Autodesk Fusion 360 part; units mm, degrees
(part 4 of 7)
  line L2251 (-109.1951, 81.084) -> (-109.1951, 80.0836)
  line L2252 (176.267, 48.0333) -> (162.267, 48.0333)
  line L2253 (200.082, 29.9838) -> (200.879, 29.9838)
  line L2254 (-109.9941, 71.1844) -> (-109.9941, 68.0838)
  line L2255 (204.329, 38.8844) -> (205.13, 38.8844)
  line L2256 (-9.983, 22.9336) -> (-9.183, 22.9336)
  line L2257 (219.132, 19.8345) -> (219.132, 14.0343)
  line L2258 (204.329, 41.9836) -> (205.13, 41.9836)
  line L2259 (224.18, 9.9333) -> (224.18, 10.9337)
  line L2260 (219.929, 14.0343) -> (219.132, 14.0343)
  line L2261 (43.205, 71.1844) -> (42.406, 71.1844)
  line L2262 (-109.9941, 68.0838) -> (-109.9941, 71.1844)
  line L2263 (223.379, 10.9337) -> (224.18, 10.9337)
  line L2264 (204.329, 14.0343) -> (205.13, 14.0343)
  line L2265 (4.817, 23.934) -> (-9.183, 23.934)
  line L2266 (200.879, 10.9337) -> (200.082, 10.9337)
  line L2267 (0.342, 28.9833) -> (14.342, 28.9833)
  line L2268 (200.879, 29.9838) -> (200.879, 33.0844)
  line L2269 (195.605, 0.1836) -> (195.605, 0.7845)
  line L2270 (219.132, 22.9336) -> (219.132, 23.934)
  line L2271 (-109.1951, 76.9844) -> (-109.1951, 71.1844)
  line L2272 (223.379, 14.0343) -> (224.18, 14.0343)
  line L2273 (-109.9941, 76.9844) -> (-109.1951, 76.9844)
  line L2274 (200.082, 10.9337) -> (200.082, 9.9333)
  line L2275 (23.867, 23.934) -> (9.867, 23.934)
  line L2276 (200.082, 9.9333) -> (200.082, 10.9337)
  line L2277 (224.18, 22.9336) -> (223.379, 22.9336)
  line L2278 (-109.1951, 80.0836) -> (-109.1951, 81.084)
  line L2279 (-109.1951, 71.1844) -> (-109.9941, 71.1844)
  line L2280 (238.182, 57.9344) -> (238.182, 52.1344)
  line L2281 (-159.2012, 33.0844) -> (-160.0019, 33.0844)
  line L2282 (224.18, 61.0336) -> (223.379, 61.0336)
  line L2283 (106.355, 71.7838) -> (106.355, 67.3134)
  line L2284 (-99.1575, 38.8844) -> (-99.1575, 41.9836)
  line L2285 (224.18, 71.1844) -> (223.379, 71.1844)
  line L2286 (205.13, 52.1344) -> (205.13, 57.9344)
  line L2287 (204.329, 52.1344) -> (204.329, 49.0338)
  line L2288 (238.182, 42.984) -> (238.182, 41.9836)
  line L2289 (104.831, 71.1844) -> (105.63, 71.1844)
  line L2290 (-23.47, 99.7592) -> (-24.269, 99.7592)
  line L2291 (244.232, 37.709) -> (244.232, 38.5083)
  line L2292 (-159.2012, 41.9836) -> (-160.0019, 41.9836)
  line L2293 (-109.9941, 99.7592) -> (-109.1951, 99.7592)
  line L2294 (186.08, 48.0333) -> (200.082, 48.0333)
  line L2295 (200.082, 48.0333) -> (186.08, 48.0333)
  line L2296 (-99.9579, 38.8844) -> (-99.9579, 33.0844)
  line L2297 (238.979, 38.8844) -> (238.182, 38.8844)
  line L2298 (-160.0019, 29.9838) -> (-159.2012, 29.9838)
  line L2299 (-159.2012, 38.8844) -> (-159.2012, 33.0844)
  line L2300 (-99.9579, 38.8844) -> (-99.1575, 38.8844)
  line L2301 (104.831, 71.7838) -> (104.831, 71.1844)
  line L2302 (-94.395, 99.7592) -> (-95.194, 99.7592)
  line L2303 (9.867, 9.9333) -> (9.867, 10.9337)
  line L2304 (223.379, 49.0338) -> (224.18, 49.0338)
  line L2305 (105.63, 71.1844) -> (105.63, 68.0838)
  line L2306 (10.449, 4.3343) -> (10.449, 3.4138)
  line L2307 (204.329, 61.0336) -> (205.13, 61.0336)
  line L2308 (16.299, 0.1836) -> (16.299, -2.6165)
  line L2309 (223.379, 68.0838) -> (224.18, 68.0838)
  line L2310 (247.333, 37.709) -> (244.232, 37.709)
  line L2311 (238.182, 38.8844) -> (238.182, 33.0844)
  line L2312 (-160.0019, 38.8844) -> (-160.0019, 41.9836)
  line L2313 (15.473, 3.4138) -> (15.473, 0.1836)
  line L2314 (106.355, 71.7838) -> (104.831, 71.7838)
  line L2315 (-159.2012, 28.9833) -> (-159.2012, 29.9838)
  line L2316 (223.379, 61.0336) -> (223.379, 57.9344)
  line L2317 (-94.9076, 38.8844) -> (-95.708, 38.8844)
  line L2318 (-159.2012, 29.9838) -> (-160.0019, 29.9838)
  line L2319 (242.482, 35.2589) -> (243.459, 35.2589)
  line L2320 (104.831, 67.0833) -> (104.831, 68.0838)
  line L2321 (113.106, 67.3134) -> (111.381, 67.3134)
  line L2322 (9.867, 14.0343) -> (9.067, 14.0343)
  line L2323 (-95.708, 38.8844) -> (-95.708, 41.9836)
  line L2324 (200.082, 62.034) -> (186.08, 62.034)
  line L2325 (186.08, 62.034) -> (200.082, 62.034)
  line L2326 (224.18, 68.0838) -> (223.379, 68.0838)
  line L2327 (-99.9579, 33.0844) -> (-99.9579, 38.8844)
  line L2328 (-160.0019, 41.9836) -> (-159.2012, 41.9836)
  line L2329 (9.867, 10.9337) -> (9.067, 10.9337)
  line L2330 (15.473, 0.1836) -> (15.473, 3.4138)
  line L2331 (113.106, 67.3134) -> (113.106, 73.5836)
  line L2332 (-24.269, 99.7592) -> (-23.47, 99.7592)
  line L2333 (-23.47, 105.5592) -> (-23.47, 99.7592)
  line L2334 (238.979, 33.0844) -> (238.979, 29.9838)
  line L2335 (-23.47, 105.5592) -> (-24.269, 105.5592)
  line L2336 (9.067, 10.9337) -> (9.067, 14.0343)
  line L2337 (242.482, 31.9583) -> (242.482, 35.2589)
  line L2338 (108.08, 67.3134) -> (106.355, 67.3134)
  line L2339 (-23.47, 108.6602) -> (-24.269, 108.6602)
  line L2340 (219.132, 52.1344) -> (219.132, 57.9344)
  line L2341 (-123.769, 49.0338) -> (-122.97, 49.0338)
  line L2342 (219.929, 49.0338) -> (219.929, 52.1344)
  line L2343 (219.132, 62.034) -> (219.132, 61.0336)
  line L2344 (-23.47, 57.9344) -> (-23.47, 52.1344)
  line L2345 (-24.271, 52.1344) -> (-23.47, 52.1344)
  line L2346 (38.156, 68.0838) -> (38.955, 68.0838)
  line L2347 (223.379, -5.0157) -> (224.18, -5.0157)
  line L2348 (219.132, 67.0833) -> (219.132, 68.0838)
  line L2349 (38.955, 76.9844) -> (38.156, 76.9844)
  line L2350 (224.18, 3.8837) -> (223.379, 3.8837)
  line L2351 (38.955, 71.1844) -> (38.156, 71.1844)
  line L2352 (219.132, 52.1344) -> (219.929, 52.1344)
  line L2353 (186.08, 61.0336) -> (185.279, 61.0336)
  line L2354 (-23.47, 49.0338) -> (-23.47, 48.0333)
  line L2355 (224.18, -9.1167) -> (224.18, -8.1163)
  line L2356 (-23.47, 48.0333) -> (-23.47, 49.0338)
  line L2357 (217.879, 3.4138) -> (216.154, 3.4138)
  line L2358 (-122.97, 61.0336) -> (-123.769, 61.0336)
  line L2359 (219.929, 71.1844) -> (219.929, 68.0838)
  line L2360 (38.156, 76.9844) -> (38.156, 71.1844)
  line L2361 (186.08, 52.1344) -> (185.279, 52.1344)
  line L2362 (219.929, 68.0838) -> (219.929, 71.1844)
  line L2363 (38.156, 71.1844) -> (38.955, 71.1844)
  line L2364 (24.155, 67.0833) -> (38.156, 67.0833)
  line L2365 (-23.47, 52.1344) -> (-24.271, 52.1344)
  line L2366 (219.132, 62.034) -> (205.13, 62.034)
  line L2367 (224.18, -8.1163) -> (223.379, -8.1163)
  line L2368 (224.18, -5.0157) -> (224.18, 0.7845)
  line L2369 (186.08, 49.0338) -> (186.08, 48.0333)
  line L2370 (223.379, 0.7845) -> (223.379, 3.8837)
  line L2371 (219.132, 71.1844) -> (219.929, 71.1844)
  line L2372 (200.082, 49.0338) -> (200.082, 48.0333)
  line L2373 (41.336, -8.1163) -> (41.336, -5.0157)
  line L2374 (-114.244, 71.1844) -> (-114.244, 76.9844)
  line L2375 (185.279, 61.0336) -> (185.279, 57.9344)
  line L2376 (185.279, 52.1344) -> (186.08, 52.1344)
  line L2377 (216.154, 3.4138) -> (217.879, 3.4138)
  line L2378 (200.082, 48.0333) -> (200.082, 49.0338)
  line L2379 (-133.808, 29.9838) -> (-133.808, 33.0844)
  line L2380 (40.537, -5.0157) -> (41.336, -5.0157)
  line L2381 (-114.244, 80.0836) -> (-113.445, 80.0836)
  line L2382 (223.379, -8.1163) -> (223.379, -5.0157)
  line L2383 (219.132, 49.0338) -> (219.132, 48.0333)
  arc A42 (183.673, 118.9832) -> (181.673, 120.9832) centre (181.673, 118.9832) ccw
  line L2384 (-133.0076, 41.9836) -> (-133.808, 41.9836)
  line L2385 (219.929, 61.0336) -> (219.929, 57.9344)
  line L2386 (176.267, 108.6602) -> (177.068, 108.6602)
  line L2387 (219.132, 49.0338) -> (219.929, 49.0338)
  line L2388 (-23.47, 62.034) -> (-23.47, 61.0336)
  line L2389 (-113.445, 76.9844) -> (-114.244, 76.9844)
  circle A43 centre (171.973, 117.5832) radius 1.7
  line L2390 (26.536, -8.1163) -> (25.737, -8.1163)
  line L2391 (224.18, -5.0157) -> (223.379, -5.0157)
  line L2392 (-27.72, 61.0336) -> (-27.72, 57.9344)
  line L2393 (-114.244, 80.0836) -> (-114.244, 81.084)
  line L2394 (-114.244, 68.0838) -> (-113.445, 68.0838)
  line L2395 (185.279, 52.1344) -> (185.279, 49.0338)
  line L2396 (-24.271, 57.9344) -> (-24.271, 61.0336)
  line L2397 (219.132, 57.9344) -> (219.132, 52.1344)
  line L2398 (186.308, 96.8822) -> (186.308, 108.8822)
  line L2399 (185.808, 109.3822) -> (198.508, 109.3822)
  line L2400 (25.737, -8.1163) -> (25.737, -5.0157)
  line L2401 (-113.445, 80.0836) -> (-113.445, 76.9844)
  line L2402 (219.132, 67.0833) -> (205.13, 67.0833)
  line L2403 (186.08, 57.9344) -> (185.279, 57.9344)
  line L2404 (-133.808, 29.9838) -> (-133.0076, 29.9838)
  line L2405 (-24.271, 49.0338) -> (-23.47, 49.0338)
  line L2406 (198.008, 96.8822) -> (186.308, 96.8822)
  line L2407 (219.132, 61.0336) -> (219.132, 62.034)
  line L2408 (185.279, 61.0336) -> (186.08, 61.0336)
  line L2409 (-24.271, 49.0338) -> (-24.271, 52.1344)
  line L2410 (-133.0076, 29.9838) -> (-133.0076, 28.9833)
  line L2411 (185.279, 49.0338) -> (186.08, 49.0338)
  line L2412 (217.879, 3.4138) -> (217.879, 0.1836)
  line L2413 (185.279, 57.9344) -> (185.279, 61.0336)
  line L2414 (219.929, 52.1344) -> (219.132, 52.1344)
  line L2415 (216.154, -8.8866) -> (216.154, -9.8664)
  line L2416 (-133.808, 41.9836) -> (-133.808, 38.8844)
  line L2417 (224.18, 0.7845) -> (223.379, 0.7845)
  line L2418 (-133.0076, 28.9833) -> (-133.0076, 29.9838)
  line L2419 (-24.271, 57.9344) -> (-23.47, 57.9344)
  line L2420 (217.879, -8.8866) -> (217.879, -2.6165)
  line L2421 (-113.445, 68.0838) -> (-114.244, 68.0838)
  line L2422 (41.336, -5.0157) -> (40.537, -5.0157)
  line L2423 (-113.445, 80.0836) -> (-114.244, 80.0836)
  line L2424 (25.737, -5.0157) -> (25.737, -8.1163)
  line L2425 (224.18, -8.1163) -> (224.18, -9.1167)
  line L2426 (-24.271, 52.1344) -> (-24.271, 49.0338)
  line L2427 (219.929, 68.0838) -> (219.132, 68.0838)
  line L2428 (30.798, -18.7426) -> (30.798, -15.9426)
  line L2429 (-114.244, 68.0838) -> (-114.244, 67.0833)
  line L2430 (-133.808, 41.9836) -> (-133.0076, 41.9836)
  line L2431 (-133.808, 38.8844) -> (-133.808, 41.9836)
  line L2432 (41.336, -5.0157) -> (41.336, -8.1163)
  line L2433 (200.082, 61.0336) -> (200.082, 62.034)
  line L2434 (186.08, 62.034) -> (186.08, 61.0336)
  line L2435 (-113.445, 71.1844) -> (-113.445, 68.0838)
  line L2436 (-114.244, 76.9844) -> (-113.445, 76.9844)
  line L2437 (172.373, 120.9832) -> (171.573, 120.9832)
  line L2438 (185.279, 57.9344) -> (186.08, 57.9344)
  line L2439 (177.068, 105.5592) -> (176.267, 105.5592)
  line L2440 (-23.47, 49.0338) -> (-24.271, 49.0338)
  line L2441 (-133.808, 33.0844) -> (-133.0076, 33.0844)
  line L2442 (-23.47, 61.0336) -> (-23.47, 62.034)
  line L2443 (216.154, 4.3343) -> (216.154, 3.4138)
  line L2444 (-133.808, 38.8844) -> (-133.0076, 38.8844)
  line L2445 (176.267, 105.5592) -> (177.068, 105.5592)
  line L2446 (176.267, 96.6592) -> (177.068, 96.6592)
  line L2447 (219.132, 68.0838) -> (219.132, 67.0833)
  line L2448 (-114.244, 81.084) -> (-114.244, 80.0836)
  line L2449 (186.08, 61.0336) -> (186.08, 62.034)
  line L2450 (-27.72, 52.1344) -> (-27.72, 49.0338)
  line L2451 (216.154, 3.4138) -> (216.154, 4.3343)
  line L2452 (26.536, -9.1167) -> (26.536, -8.1163)
  line L2453 (205.13, 62.034) -> (219.132, 62.034)
  line L2454 (40.537, -9.1167) -> (26.536, -9.1167)
  line L2455 (-113.445, 68.0838) -> (-113.445, 71.1844)
  line L2456 (26.536, -9.1167) -> (40.537, -9.1167)
  line L2457 (219.132, 68.0838) -> (219.929, 68.0838)
  line L2458 (-133.0076, 42.984) -> (-133.0076, 41.9836)
  line L2459 (-23.47, 52.1344) -> (-23.47, 57.9344)
  line L2460 (219.132, 48.0333) -> (219.132, 49.0338)
  line L2461 (-113.445, 71.1844) -> (-114.244, 71.1844)
  line L2462 (-144.4011, 33.0844) -> (-144.4011, 29.9838)
  line L2463 (-133.0076, 41.9836) -> (-133.0076, 42.984)
  line L2464 (186.08, 48.0333) -> (186.08, 49.0338)
  line L2465 (14.63, 49.0338) -> (14.63, 48.0333)
  line L2466 (-113.445, 76.9844) -> (-113.445, 80.0836)
  line L2467 (176.267, 105.5592) -> (176.267, 99.7592)
  line L2468 (223.379, 3.8837) -> (223.379, 0.7845)
  line L2469 (-27.72, 57.9344) -> (-27.72, 61.0336)
  line L2470 (177.068, 108.6602) -> (177.068, 105.5592)
  line L2471 (-27.72, 49.0338) -> (-27.72, 52.1344)
  line L2472 (9.581, 61.0336) -> (10.38, 61.0336)
  line L2473 (219.929, 52.1344) -> (219.929, 49.0338)
  line L2474 (224.18, 4.8841) -> (224.18, 3.8837)
  line L2475 (205.13, 67.0833) -> (219.132, 67.0833)
  line L2476 (186.08, 52.1344) -> (186.08, 57.9344)
  line L2477 (-114.244, 67.0833) -> (-114.244, 68.0838)
  line L2478 (185.279, 49.0338) -> (185.279, 52.1344)
  line L2479 (-133.808, 33.0844) -> (-133.808, 29.9838)
  line L2480 (186.08, 57.9344) -> (186.08, 52.1344)
  line L2481 (176.267, 96.6592) -> (176.267, 95.6582)
  line L2482 (40.537, -9.1167) -> (40.537, -8.1163)
  line L2483 (-114.244, 76.9844) -> (-114.244, 71.1844)
  line L2484 (223.379, -8.1163) -> (224.18, -8.1163)
  line L2485 (-23.47, 57.9344) -> (-24.271, 57.9344)
  line L2486 (186.08, 49.0338) -> (185.279, 49.0338)
  line L2487 (198.008, 108.8822) -> (198.008, 96.8822)
  line L2488 (216.154, -8.8866) -> (217.879, -8.8866)
  line L2489 (41.336, -8.1163) -> (40.537, -8.1163)
  line L2490 (176.267, 99.7592) -> (176.267, 105.5592)
  line L2491 (-24.271, 61.0336) -> (-24.271, 57.9344)
  line L2492 (13.831, 57.9344) -> (14.63, 57.9344)
  line L2493 (219.929, 57.9344) -> (219.929, 61.0336)
  line L2494 (-24.271, 61.0336) -> (-23.47, 61.0336)
  line L2495 (177.068, 99.7592) -> (176.267, 99.7592)
  line L2496 (177.068, 96.6592) -> (177.068, 99.7592)
  line L2497 (217.879, -2.6165) -> (218.705, -2.6165)
  line L2498 (-133.0076, 29.9838) -> (-133.808, 29.9838)
  line L2499 (-118.7201, 48.0333) -> (-104.719, 48.0333)
  line L2500 (9.581, 57.9344) -> (10.38, 57.9344)
  line L2501 (26.536, -5.0157) -> (25.737, -5.0157)
  line L2502 (-23.47, 61.0336) -> (-24.271, 61.0336)
  line L2503 (219.929, 71.1844) -> (219.132, 71.1844)
  line L2504 (-114.244, 71.1844) -> (-113.445, 71.1844)
  line L2505 (219.929, 57.9344) -> (219.132, 57.9344)
  line L2506 (200.082, 57.9344) -> (200.082, 52.1344)
  line L2507 (-133.0076, 33.0844) -> (-133.808, 33.0844)
  line L2508 (218.705, -2.6165) -> (217.879, -2.6165)
  line L2509 (10.38, 52.1344) -> (10.38, 49.0338)
  arc A44 (28.798, -20.7426) -> (30.798, -18.7426) centre (28.798, -18.7426) ccw
  line L2510 (224.18, 3.8837) -> (224.18, 4.8841)
  line L2511 (-104.719, 48.0333) -> (-118.7201, 48.0333)
  line L2512 (-144.4011, 41.9836) -> (-144.4011, 38.8844)
  line L2513 (-144.4011, 38.8844) -> (-144.4011, 41.9836)
  line L2514 (219.132, 57.9344) -> (219.929, 57.9344)
  line L2515 (219.132, 61.0336) -> (219.929, 61.0336)
  line L2516 (10.38, 52.1344) -> (9.581, 52.1344)
  line L2517 (14.63, 52.1344) -> (13.831, 52.1344)
  arc A45 (183.673, 116.1832) -> (185.673, 114.1832) centre (185.673, 116.1832) ccw
  arc A46 (32.798, -13.9426) -> (30.798, -15.9426) centre (32.798, -15.9426) ccw
  line L2518 (223.379, -5.0157) -> (223.379, -8.1163)
  line L2519 (40.537, -8.1163) -> (41.336, -8.1163)
  line L2520 (177.068, 108.6602) -> (176.267, 108.6602)
  line L2521 (-133.0076, 38.8844) -> (-133.808, 38.8844)
  line L2522 (183.673, 118.9832) -> (183.673, 116.1832)
  line L2523 (-104.719, 62.034) -> (-118.7201, 62.034)
  line L2524 (14.63, 52.1344) -> (14.63, 57.9344)
  line L2525 (13.831, 52.1344) -> (14.63, 52.1344)
  circle A47 centre (171.973, 117.5832) radius 1.7
  line L2526 (219.929, 61.0336) -> (219.132, 61.0336)
  line L2527 (25.737, -8.1163) -> (26.536, -8.1163)
  line L2528 (205.13, 48.0333) -> (219.132, 48.0333)
  line L2529 (217.879, -8.8866) -> (216.154, -8.8866)
  line L2530 (-118.7201, 62.034) -> (-104.719, 62.034)
  line L2531 (218.705, 0.1836) -> (217.879, 0.1836)
  line L2532 (185.808, 96.3822) -> (185.808, 109.3822)
  line L2533 (217.879, 0.1836) -> (217.879, 3.4138)
  line L2534 (10.38, 49.0338) -> (9.581, 49.0338)
  line L2535 (-133.0076, 38.8844) -> (-133.0076, 33.0844)
  line L2536 (9.581, 62.034) -> (9.581, 61.0336)
  line L2537 (-133.0076, 33.0844) -> (-133.0076, 38.8844)
  line L2538 (25.737, -5.0157) -> (26.536, -5.0157)
  line L2539 (26.536, -8.1163) -> (26.536, -9.1167)
  line L2540 (200.082, 52.1344) -> (200.879, 52.1344)
  line L2541 (224.18, 0.7845) -> (224.18, -5.0157)
  line L2542 (40.537, -5.0157) -> (40.537, 0.7845)
  line L2543 (217.879, -2.6165) -> (217.879, -8.8866)
  line L2544 (-144.4011, 29.9838) -> (-144.4011, 33.0844)
  line L2545 (218.705, 0.1836) -> (218.705, -2.6165)
  line L2546 (198.508, 96.3822) -> (185.808, 96.3822)
  line L2547 (9.581, 48.0333) -> (9.581, 49.0338)
  line L2548 (223.379, 0.7845) -> (224.18, 0.7845)
  line L2549 (13.831, 57.9344) -> (13.831, 61.0336)
  line L2550 (-142.5325, 23.934) -> (-142.5325, 22.9336)
  line L2551 (26.536, 0.7845) -> (26.536, -5.0157)
  line L2552 (218.705, -2.6165) -> (218.705, 0.1836)
  line L2553 (177.068, 99.7592) -> (177.068, 96.6592)
  line L2554 (-142.5325, 22.9336) -> (-142.5325, 23.934)
  line L2555 (40.537, -8.1163) -> (40.537, -9.1167)
  line L2556 (9.581, 49.0338) -> (10.38, 49.0338)
  line L2557 (223.379, 3.8837) -> (224.18, 3.8837)
  line L2558 (176.267, 95.6582) -> (176.267, 96.6592)
  line L2559 (40.537, 0.7845) -> (40.537, -5.0157)
  line L2560 (26.536, -5.0157) -> (26.536, 0.7845)
  line L2561 (204.329, 52.1344) -> (205.13, 52.1344)
  line L2562 (186.308, 108.8822) -> (198.008, 108.8822)
  line L2563 (13.831, 61.0336) -> (14.63, 61.0336)
  line L2564 (216.154, -9.8664) -> (216.154, -8.8866)
  line L2565 (14.63, 48.0333) -> (14.63, 49.0338)
  line L2566 (205.13, 49.0338) -> (205.13, 48.0333)
  line L2567 (-143.3331, 19.8345) -> (-142.5325, 19.8345)
  line L2568 (10.38, 57.9344) -> (9.581, 57.9344)
  line L2569 (-109.1951, 95.6582) -> (-95.194, 95.6582)
  line L2570 (-90.1451, 96.6592) -> (-90.9441, 96.6592)
  line L2571 (223.379, 49.0338) -> (223.379, 52.1344)
  line L2572 (200.082, 62.034) -> (200.082, 61.0336)
  line L2573 (200.082, 49.0338) -> (200.879, 49.0338)
  line L2574 (-109.9941, 99.7592) -> (-109.9941, 96.6592)
  line L2575 (205.13, 48.0333) -> (205.13, 49.0338)
  line L2576 (-143.3331, 22.9336) -> (-143.3331, 19.8345)
  line L2577 (-143.3331, 19.8345) -> (-143.3331, 22.9336)
  line L2578 (177.068, 96.6592) -> (176.267, 96.6592)
  line L2579 (-90.1451, 96.6592) -> (-90.1451, 95.6582)
  line L2580 (198.508, 109.3822) -> (198.508, 96.3822)
  line L2581 (205.13, 61.0336) -> (204.329, 61.0336)
  line L2582 (13.831, 61.0336) -> (13.831, 57.9344)
  line L2583 (224.18, 67.0833) -> (224.18, 68.0838)
  line L2584 (217.879, 0.1836) -> (218.705, 0.1836)
  line L2585 (-142.5325, 19.8345) -> (-143.3331, 19.8345)
  line L2586 (200.879, 57.9344) -> (200.879, 61.0336)
  line L2587 (-90.9441, 99.7592) -> (-90.9441, 96.6592)
  line L2588 (-142.5325, 22.9336) -> (-143.3331, 22.9336)
  line L2589 (176.267, 108.6602) -> (176.267, 109.6602)
  line L2590 (177.068, 105.5592) -> (177.068, 108.6602)
  line L2591 (200.879, 57.9344) -> (200.082, 57.9344)
  line L2592 (-109.9941, 96.6592) -> (-109.9941, 99.7592)
  line L2593 (205.13, 57.9344) -> (205.13, 52.1344)
  line L2594 (224.18, 57.9344) -> (224.18, 52.1344)
  line L2595 (-143.3331, 22.9336) -> (-142.5325, 22.9336)
  line L2596 (223.379, 61.0336) -> (224.18, 61.0336)
  line L2597 (205.13, 52.1344) -> (204.329, 52.1344)
  line L2598 (223.379, 57.9344) -> (224.18, 57.9344)
  line L2599 (224.18, 52.1344) -> (224.18, 57.9344)
  line L2600 (224.18, 61.0336) -> (224.18, 62.034)
  line L2601 (223.379, 71.1844) -> (223.379, 68.0838)
  line L2602 (204.329, 57.9344) -> (205.13, 57.9344)
  line L2603 (200.879, 52.1344) -> (200.082, 52.1344)
  line L2604 (223.379, 68.0838) -> (223.379, 71.1844)
  line L2605 (204.329, 57.9344) -> (204.329, 61.0336)
  line L2606 (-94.395, 99.7592) -> (-94.395, 96.6592)
  line L2607 (9.067, 14.0343) -> (9.067, 10.9337)
  line L2608 (224.18, 49.0338) -> (224.18, 48.0333)
  line L2609 (205.13, 62.034) -> (205.13, 61.0336)
  line L2610 (162.267, 109.6602) -> (176.267, 109.6602)
  line L2611 (-90.1451, 99.7592) -> (-90.9441, 99.7592)
  line L2612 (223.379, 52.1344) -> (223.379, 49.0338)
  line L2613 (204.329, 61.0336) -> (204.329, 57.9344)
  line L2614 (181.673, 120.9832) -> (162.273, 120.9832)
  line L2615 (-90.9441, 99.7592) -> (-90.1451, 99.7592)
  line L2616 (-95.194, 95.6582) -> (-109.1951, 95.6582)
  line L2617 (162.267, 95.6582) -> (176.267, 95.6582)
  line L2618 (13.748, 3.4138) -> (15.473, 3.4138)
  line L2619 (204.329, 49.0338) -> (205.13, 49.0338)
  line L2620 (176.267, 109.6602) -> (176.267, 108.6602)
  line L2621 (-94.395, 96.6592) -> (-94.395, 99.7592)
  line L2622 (-95.194, 96.6592) -> (-94.395, 96.6592)
  line L2623 (176.267, 99.7592) -> (177.068, 99.7592)
  line L2624 (200.879, 52.1344) -> (200.879, 49.0338)
  line L2625 (-109.1951, 96.6592) -> (-109.1951, 95.6582)
  line L2626 (-90.1451, 95.6582) -> (-90.1451, 96.6592)
  line L2627 (224.18, 68.0838) -> (224.18, 67.0833)
  line L2628 (200.082, 61.0336) -> (200.879, 61.0336)
  line L2629 (243.459, 36.984) -> (243.459, 35.2589)
  line L2630 (224.18, 62.034) -> (224.18, 61.0336)
  line L2631 (-160.0019, 29.9838) -> (-160.0019, 33.0844)
  line L2632 (205.13, 57.9344) -> (204.329, 57.9344)
  line L2633 (-160.0019, 41.9836) -> (-160.0019, 38.8844)
  line L2634 (238.182, 52.1344) -> (238.182, 57.9344)
  line L2635 (200.082, 52.1344) -> (200.082, 57.9344)
  line L2636 (-95.194, 95.6582) -> (-95.194, 96.6592)
  line L2637 (223.379, 57.9344) -> (223.379, 61.0336)
  line L2638 (244.232, 38.5083) -> (244.232, 37.709)
  line L2639 (111.381, 67.3134) -> (113.106, 67.3134)
  line L2640 (224.18, 52.1344) -> (223.379, 52.1344)
  line L2641 (200.879, 49.0338) -> (200.879, 52.1344)
  line L2642 (200.879, 61.0336) -> (200.082, 61.0336)
  line L2643 (205.13, 61.0336) -> (205.13, 62.034)
  line L2644 (243.23, 38.5083) -> (244.232, 38.5083)
  line L2645 (-109.9941, 96.6592) -> (-109.1951, 96.6592)
  line L2646 (238.182, 48.0333) -> (238.182, 49.0338)
  line L2647 (16.299, 0.1836) -> (15.473, 0.1836)
  line L2648 (-90.9441, 96.6592) -> (-90.9441, 99.7592)
  line L2649 (-159.2012, 42.984) -> (-159.2012, 41.9836)
  line L2650 (-95.194, 99.7592) -> (-94.395, 99.7592)
  line L2651 (113.106, 73.5836) -> (113.106, 67.3134)
  line L2652 (105.63, 68.0838) -> (105.63, 71.1844)
  line L2653 (205.13, 49.0338) -> (204.329, 49.0338)
  line L2654 (200.082, 57.9344) -> (200.879, 57.9344)
  line L2655 (-109.1951, 99.7592) -> (-109.9941, 99.7592)
  line L2656 (224.18, 57.9344) -> (223.379, 57.9344)
  line L2657 (238.182, 28.9833) -> (238.182, 29.9838)
  line L2658 (238.182, 33.0844) -> (238.979, 33.0844)
  line L2659 (-159.2012, 38.8844) -> (-160.0019, 38.8844)
  line L2660 (-95.194, 96.6592) -> (-95.194, 95.6582)
  line L2661 (9.067, 14.0343) -> (9.867, 14.0343)
  line L2662 (223.379, 71.1844) -> (224.18, 71.1844)
  line L2663 (243.459, 35.2589) -> (243.459, 36.984)
  line L2664 (-160.0019, 33.0844) -> (-159.2012, 33.0844)
  line L2665 (-90.9441, 96.6592) -> (-90.1451, 96.6592)
  line L2666 (13.748, 3.4138) -> (13.748, 4.3343)
  line L2667 (-160.0019, 33.0844) -> (-160.0019, 29.9838)
  line L2668 (-109.1951, 95.6582) -> (-109.1951, 96.6592)
  line L2669 (247.929, 36.984) -> (243.459, 36.984)
  line L2670 (224.18, 48.0333) -> (224.18, 49.0338)
  line L2671 (242.482, 35.2589) -> (242.482, 31.9583)
  line L2672 (200.879, 61.0336) -> (200.879, 57.9344)
  line L2673 (111.381, 67.3134) -> (111.381, 66.3337)
  line L2674 (238.979, 29.9838) -> (238.979, 33.0844)
  line L2675 (200.879, 49.0338) -> (200.082, 49.0338)
  line L2676 (238.182, 38.8844) -> (238.979, 38.8844)
  line L2677 (-94.395, 96.6592) -> (-95.194, 96.6592)
  line L2678 (224.18, 49.0338) -> (223.379, 49.0338)
  line L2679 (15.473, 3.4138) -> (13.748, 3.4138)
  line L2680 (106.355, 67.3134) -> (106.355, 71.7838)
  line L2681 (223.379, 52.1344) -> (224.18, 52.1344)
  line L2682 (108.08, 66.3337) -> (108.08, 67.3134)
  line L2683 (-159.2012, 29.9838) -> (-159.2012, 28.9833)
  line L2684 (204.329, 49.0338) -> (204.329, 52.1344)
  line L2685 (13.748, 4.3343) -> (13.748, 3.4138)
  line L2686 (-159.2012, 33.0844) -> (-159.2012, 38.8844)
  line L2687 (-109.1951, 96.6592) -> (-109.9941, 96.6592)
  line L2688 (15.473, 0.1836) -> (16.299, 0.1836)
  line L2689 (108.08, 67.3134) -> (108.08, 66.3337)
  line L2690 (-160.0019, 38.8844) -> (-159.2012, 38.8844)
  line L2691 (253.129, 38.5083) -> (252.529, 38.5083)
  line L2692 (252.529, 29.4092) -> (249.732, 29.4092)
  line L2693 (-42.52, 108.6602) -> (-43.319, 108.6602)
  line L2694 (15.473, -8.8866) -> (15.473, -2.6165)
  line L2695 (247.333, 52.509) -> (247.333, 53.3084)
  line L2696 (-145.2017, 38.8844) -> (-145.2017, 33.0844)
  line L2697 (-42.52, 96.6592) -> (-42.52, 95.6582)
  line L2698 (-95.194, 99.7592) -> (-95.194, 105.5592)
  line L2699 (252.529, 52.509) -> (253.129, 52.509)
  line L2700 (-43.319, 105.5592) -> (-42.52, 105.5592)
  line L2701 (-145.2017, 42.984) -> (-145.2017, 41.9836)
  line L2702 (257.232, 38.5083) -> (256.23, 38.5083)
  line L2703 (-43.321, 57.9344) -> (-43.321, 61.0336)
  line L2704 (-109.1951, 108.6602) -> (-109.1951, 109.6602)
  line L2705 (-42.52, 48.0333) -> (-42.52, 49.0338)
  line L2706 (-42.52, 49.0338) -> (-42.52, 48.0333)
  line L2707 (-145.2017, 41.9836) -> (-145.2017, 42.984)
  line L2708 (-42.52, 105.5592) -> (-42.52, 99.7592)
  line L2709 (249.732, 29.4092) -> (249.732, 30.2332)
  line L2710 (244.232, 52.509) -> (244.232, 53.3084)
  line L2711 (247.333, 53.3084) -> (247.333, 52.509)
  line L2712 (113.106, 76.3836) -> (113.106, 79.6137)
  line L2713 (-90.1451, 108.6602) -> (-90.9441, 108.6602)
  line L2714 (-42.52, 96.6592) -> (-43.319, 96.6592)
  line L2715 (-95.194, 108.6602) -> (-95.194, 109.6602)
  line L2716 (-43.319, 96.6592) -> (-42.52, 96.6592)
  line L2717 (113.106, 79.6137) -> (111.381, 79.6137)
  line L2718 (113.93, 76.3836) -> (113.106, 76.3836)
  line L2719 (243.459, 54.0334) -> (247.929, 54.0334)
  line L2720 (-90.1451, 105.5592) -> (-90.1451, 99.7592)
  line L2721 (106.355, 79.6137) -> (108.08, 79.6137)
  line L2722 (-42.52, 61.0336) -> (-42.52, 62.034)
  line L2723 (-145.2017, 29.9838) -> (-144.4011, 29.9838)
  line L2724 (105.63, 80.0836) -> (104.831, 80.0836)
  line L2725 (106.355, 76.3836) -> (104.831, 76.3836)
  line L2726 (-46.77, 57.9344) -> (-46.77, 61.0336)
  line L2727 (244.232, 53.3084) -> (247.333, 53.3084)
  line L2728 (-109.1951, 99.7592) -> (-109.1951, 105.5592)
  line L2729 (-145.2017, 28.9833) -> (-159.2012, 28.9833)
  line L2730 (-90.4329, 22.9336) -> (-90.4329, 23.934)
  line L2731 (255.761, 36.984) -> (255.761, 35.2589)
  line L2732 (-104.4326, 23.934) -> (-90.4329, 23.934)
  line L2733 (-43.319, 108.6602) -> (-43.319, 105.5592)
  line L2734 (-90.1451, 99.7592) -> (-90.1451, 105.5592)
  line L2735 (243.459, 55.7585) -> (242.482, 55.7585)
  line L2736 (252.529, 30.2332) -> (252.529, 29.4092)
  line L2737 (-144.4011, 41.9836) -> (-145.2017, 41.9836)
  line L2738 (-46.77, 52.1344) -> (-47.569, 52.1344)
  line L2739 (253.129, 38.5083) -> (253.129, 37.709)
  line L2740 (-145.2017, 38.8844) -> (-144.4011, 38.8844)
  line L2741 (-105.233, 22.9336) -> (-104.4326, 22.9336)
  line L2742 (252.529, 38.5083) -> (252.529, 36.984)
  line L2743 (-46.77, 61.0336) -> (-47.569, 61.0336)
  line L2744 (105.63, 76.9844) -> (104.831, 76.9844)
  line L2745 (113.93, 76.3836) -> (113.93, 73.5836)
  line L2746 (-145.2017, 41.9836) -> (-144.4011, 41.9836)
  line L2747 (-42.52, 99.7592) -> (-42.52, 105.5592)
  line L2748 (244.232, 52.509) -> (243.23, 52.509)
  line L2749 (-28.519, 109.6602) -> (-42.52, 109.6602)
  line L2750 (-95.194, 105.5592) -> (-95.194, 99.7592)
  line L2751 (-43.321, 61.0336) -> (-43.321, 57.9344)
  line L2752 (-46.77, 52.1344) -> (-46.77, 49.0338)
  line L2753 (256.681, 35.2589) -> (255.761, 35.2589)
  line L2754 (256.23, 38.5083) -> (257.232, 38.5083)
  line L2755 (-28.519, 99.7592) -> (-28.519, 105.5592)
  line L2756 (-46.77, 49.0338) -> (-47.569, 49.0338)
  line L2757 (-109.1951, 105.5592) -> (-109.1951, 99.7592)
  line L2758 (252.529, 54.0334) -> (252.529, 52.509)
  line L2759 (-28.519, 95.6582) -> (-42.52, 95.6582)
  line L2760 (-28.519, 108.6602) -> (-28.519, 109.6602)
  line L2761 (-89.6325, 19.8345) -> (-89.6325, 22.9336)
  line L2762 (256.23, 52.509) -> (257.232, 52.509)
  line L2763 (-104.4326, 23.934) -> (-104.4326, 22.9336)
  line L2764 (105.63, 80.0836) -> (105.63, 76.9844)
  line L2765 (104.831, 80.0836) -> (105.63, 80.0836)
  line L2766 (200.082, 68.0838) -> (200.082, 67.0833)
  line L2767 (256.23, 37.709) -> (256.23, 38.5083)
  line L2768 (-104.4326, 22.9336) -> (-104.4326, 23.934)
  line L2769 (247.929, 52.509) -> (247.333, 52.509)
  line L2770 (-89.6325, 22.9336) -> (-89.6325, 19.8345)
  line L2771 (200.879, 76.9844) -> (200.879, 80.0836)
  line L2772 (255.761, 55.7585) -> (256.681, 55.7585)
  line L2773 (-47.569, 52.1344) -> (-47.569, 57.9344)
  line L2774 (205.13, 81.084) -> (205.13, 80.0836)
  line L2775 (-159.2012, 42.984) -> (-145.2017, 42.984)
  line L2776 (247.333, 52.509) -> (247.929, 52.509)
  line L2777 (104.831, 76.3836) -> (106.355, 76.3836)
  line L2778 (252.529, 36.984) -> (255.761, 36.984)
  line L2779 (205.13, 71.1844) -> (204.329, 71.1844)
  line L2780 (104.831, 76.9844) -> (105.63, 76.9844)
  line L2781 (238.182, 9.9333) -> (224.18, 9.9333)
  line L2782 (-42.52, 95.6582) -> (-28.519, 95.6582)
  line L2783 (-28.519, 108.6602) -> (-27.72, 108.6602)
  line L2784 (255.761, 54.0334) -> (255.761, 55.7585)
  line L2785 (243.23, 52.509) -> (244.232, 52.509)
  line L2786 (-9.183, 9.9333) -> (4.817, 9.9333)
  line L2787 (-105.233, 22.9336) -> (-105.233, 19.8345)
  line L2788 (205.13, 68.0838) -> (204.329, 68.0838)
  line L2789 (-47.569, 61.0336) -> (-46.77, 61.0336)
  line L2790 (106.355, 79.6137) -> (106.355, 76.3836)
  line L2791 (113.106, 76.3836) -> (113.93, 76.3836)
  line L2792 (238.182, 23.934) -> (224.18, 23.934)
  line L2793 (256.23, 53.3084) -> (253.129, 53.3084)
  line L2794 (255.761, 30.2332) -> (252.529, 30.2332)
  line L2795 (-28.519, 96.6592) -> (-28.519, 95.6582)
  line L2796 (205.13, 67.0833) -> (205.13, 68.0838)
  line L2797 (256.681, 35.2589) -> (256.681, 31.9583)
  line L2798 (-27.72, 96.6592) -> (-28.519, 96.6592)
  line L2799 (256.23, 37.709) -> (253.129, 37.709)
  line L2800 (256.23, 52.509) -> (256.23, 53.3084)
  line L2801 (247.333, 38.5083) -> (247.333, 37.709)
  line L2802 (-42.52, 57.9344) -> (-43.321, 57.9344)
  line L2803 (200.082, 76.9844) -> (200.082, 71.1844)
  line L2804 (204.329, 71.1844) -> (204.329, 68.0838)
  line L2805 (-42.52, 57.9344) -> (-42.52, 52.1344)
  line L2806 (-104.4326, 22.9336) -> (-105.233, 22.9336)
  line L2807 (204.329, 76.9844) -> (205.13, 76.9844)
  line L2808 (253.129, 52.509) -> (253.129, 53.3084)
  line L2809 (-43.321, 57.9344) -> (-42.52, 57.9344)
  line L2810 (252.529, 36.984) -> (252.529, 38.5083)
  line L2811 (238.182, 4.8841) -> (224.18, 4.8841)
  line L2812 (200.879, 76.9844) -> (200.082, 76.9844)
  line L2813 (-9.183, 10.9337) -> (-9.183, 9.9333)
  line L2814 (-47.569, 57.9344) -> (-46.77, 57.9344)
  line L2815 (247.929, 54.0334) -> (247.929, 52.509)
  line L2816 (-113.445, 99.7592) -> (-113.445, 96.6592)
  line L2817 (205.13, 76.9844) -> (204.329, 76.9844)
  line L2818 (252.529, 52.509) -> (252.529, 54.0334)
  line L2819 (224.18, 4.8841) -> (238.182, 4.8841)
  line L2820 (4.817, 14.0343) -> (5.618, 14.0343)
  line L2821 (205.13, 80.0836) -> (205.13, 81.084)
  line L2822 (243.459, 54.0334) -> (243.459, 55.7585)
  line L2823 (204.329, 76.9844) -> (204.329, 80.0836)
  line L2824 (-90.4329, 23.934) -> (-90.4329, 22.9336)
  line L2825 (255.761, 30.2332) -> (255.761, 31.9583)
  line L2826 (255.761, 55.7585) -> (255.761, 54.0334)
  line L2827 (-42.52, 62.034) -> (-42.52, 61.0336)
  line L2828 (-114.244, 96.6592) -> (-114.244, 95.6582)
  line L2829 (-28.519, 109.6602) -> (-28.519, 108.6602)
  line L2830 (-104.4326, 19.8345) -> (-105.233, 19.8345)
  line L2831 (200.082, 68.0838) -> (200.879, 68.0838)
  line L2832 (-114.244, 95.6582) -> (-114.244, 96.6592)
  line L2833 (-114.244, 99.7592) -> (-114.244, 105.5592)
  line L2834 (-47.569, 49.0338) -> (-47.569, 48.0333)
  line L2835 (-90.4329, 19.8345) -> (-89.6325, 19.8345)
  line L2836 (-128.2451, 109.6602) -> (-114.244, 109.6602)
  line L2837 (-114.244, 108.6602) -> (-114.244, 109.6602)
  line L2838 (256.681, 31.9583) -> (256.681, 35.2589)
  arc A48 (7.398, -15.9426) -> (5.398, -13.9426) centre (5.398, -15.9426) ccw
  line L2839 (247.929, 38.5083) -> (247.333, 38.5083)
  line L2840 (-27.72, 108.6602) -> (-28.519, 108.6602)
  line L2841 (-43.321, 49.0338) -> (-42.52, 49.0338)
  line L2842 (-38.044, 81.084) -> (-52.045, 81.084)
  line L2843 (-89.6325, 19.8345) -> (-90.4329, 19.8345)
  line L2844 (-113.445, 96.6592) -> (-113.445, 99.7592)
  line L2845 (23.867, 19.8345) -> (23.867, 14.0343)
  line L2846 (257.232, 38.5083) -> (257.232, 52.509)
  line L2847 (257.232, 52.509) -> (257.232, 38.5083)
  line L2848 (-13.432, 10.9337) -> (-13.432, 14.0343)
  line L2849 (-61.57, 48.0333) -> (-47.569, 48.0333)
  line L2850 (255.761, 31.9583) -> (256.681, 31.9583)
  line L2851 (-105.233, 19.8345) -> (-104.4326, 19.8345)
  line L2852 (243.23, 38.5083) -> (243.23, 52.509)
  line L2853 (-89.6325, 22.9336) -> (-90.4329, 22.9336)
  line L2854 (-140.9519, -8.1163) -> (-140.9519, -5.0157)
  line L2855 (200.082, 71.1844) -> (200.082, 76.9844)
  line L2856 (-47.569, 57.9344) -> (-47.569, 52.1344)
  line L2857 (204.329, 68.0838) -> (204.329, 71.1844)
  line L2858 (-113.445, 108.6602) -> (-114.244, 108.6602)
  line L2859 (-42.52, 109.6602) -> (-28.519, 109.6602)
  line L2860 (-28.519, 105.5592) -> (-27.72, 105.5592)
  line L2861 (-42.52, 49.0338) -> (-43.321, 49.0338)
  line L2862 (-28.519, 99.7592) -> (-27.72, 99.7592)
  line L2863 (247.333, 37.709) -> (247.333, 38.5083)
  line L2864 (253.129, 37.709) -> (253.129, 38.5083)
  line L2865 (-140.9519, 3.8837) -> (-140.9519, 0.7845)
  line L2866 (204.329, 80.0836) -> (204.329, 76.9844)
  line L2867 (-113.445, 108.6602) -> (-113.445, 105.5592)
  line L2868 (4.817, 10.9337) -> (5.618, 10.9337)
  line L2869 (253.129, 52.509) -> (252.529, 52.509)
  line L2870 (-46.77, 57.9344) -> (-47.569, 57.9344)
  line L2871 (-140.1512, -5.0157) -> (-140.1512, 0.7845)
  line L2872 (253.129, 37.709) -> (256.23, 37.709)
  line L2873 (-9.983, 14.0343) -> (-9.183, 14.0343)
  line L2874 (-94.9076, 33.0844) -> (-95.708, 33.0844)
  line L2875 (238.979, 33.0844) -> (238.182, 33.0844)
  line L2876 (238.182, 29.9838) -> (238.182, 28.9833)
  line L2877 (-24.269, 99.7592) -> (-24.269, 96.6592)
  line L2878 (244.232, 37.709) -> (247.333, 37.709)
  line L2879 (13.748, 4.3343) -> (10.449, 4.3343)
  line L2880 (8.724, 3.4138) -> (8.724, 0.1836)
  line L2881 (113.93, 73.5836) -> (113.106, 73.5836)
  line L2882 (10.449, 3.4138) -> (8.724, 3.4138)
  line L2883 (8.724, 3.4138) -> (10.449, 3.4138)
  line L2884 (-24.269, 105.5592) -> (-24.269, 108.6602)
  line L2885 (-99.9579, 42.984) -> (-99.9579, 41.9836)
  line L2886 (243.459, 31.9583) -> (242.482, 31.9583)
  line L2887 (9.867, 10.9337) -> (9.867, 9.9333)
  line L2888 (104.831, 71.7838) -> (106.355, 71.7838)
  line L2889 (-159.2012, 41.9836) -> (-159.2012, 42.984)
  line L2890 (-99.1575, 33.0844) -> (-99.9579, 33.0844)
  line L2891 (105.63, 71.1844) -> (104.831, 71.1844)
  line L2892 (-24.269, 96.6592) -> (-24.269, 99.7592)
  line L2893 (238.979, 49.0338) -> (238.182, 49.0338)
  line L2894 (238.979, 38.8844) -> (238.979, 41.9836)
  line L2895 (238.182, 49.0338) -> (238.182, 48.0333)
  line L2896 (104.831, 68.0838) -> (105.63, 68.0838)
  line L2897 (-95.708, 33.0844) -> (-95.708, 29.9838)
  line L2898 (-23.47, 95.6582) -> (-23.47, 96.6592)
  line L2899 (-27.72, 99.7592) -> (-27.72, 96.6592)
  line L2900 (238.182, 49.0338) -> (238.979, 49.0338)
  line L2901 (111.381, 66.3337) -> (108.08, 66.3337)
  line L2902 (113.106, 73.5836) -> (113.93, 73.5836)
  line L2903 (-99.9579, 29.9838) -> (-99.9579, 28.9833)
  line L2904 (-164.763, 19.8345) -> (-163.9637, 19.8345)
  line L2905 (-94.395, 108.6602) -> (-94.395, 105.5592)
  line L2906 (243.459, 36.984) -> (247.929, 36.984)
  line L2907 (-99.9579, 41.9836) -> (-99.1575, 41.9836)
  line L2908 (108.08, 66.3337) -> (111.381, 66.3337)
  line L2909 (104.831, 71.1844) -> (104.831, 71.7838)
  line L2910 (238.979, 41.9836) -> (238.182, 41.9836)
  line L2911 (15.473, -2.6165) -> (16.299, -2.6165)
  line L2912 (238.979, 49.0338) -> (238.979, 52.1344)
  line L2913 (-163.9637, 22.9336) -> (-164.763, 22.9336)
  line L2914 (-23.47, 96.6592) -> (-24.269, 96.6592)
  line L2915 (-90.9441, 105.5592) -> (-90.9441, 108.6602)
  line L2916 (8.724, 0.1836) -> (8.724, 3.4138)
  line L2917 (238.182, 29.9838) -> (238.979, 29.9838)
  line L2918 (-27.72, 105.5592) -> (-27.72, 108.6602)
  line L2919 (104.831, 68.0838) -> (104.831, 67.0833)
  line L2920 (-24.269, 108.6602) -> (-24.269, 105.5592)
  line L2921 (242.482, 31.9583) -> (243.459, 31.9583)
  line L2922 (-99.1575, 38.8844) -> (-99.9579, 38.8844)
  line L2923 (10.449, 4.3343) -> (13.748, 4.3343)
  circle A49 centre (-94.901, 117.5832) radius 1.7
  line L2924 (-94.9076, 41.9836) -> (-95.708, 41.9836)
  line L2925 (-94.9076, 28.9833) -> (-94.9076, 29.9838)
  line L2926 (10.449, 3.4138) -> (10.449, 4.3343)
  line L2927 (-27.72, 96.6592) -> (-27.72, 99.7592)
  line L2928 (238.979, 52.1344) -> (238.979, 49.0338)
  line L2929 (-109.9941, 108.6602) -> (-109.9941, 105.5592)
  line L2930 (106.355, 67.3134) -> (108.08, 67.3134)
  line L2931 (186.08, 68.0838) -> (186.08, 67.0833)
  line L2932 (-95.708, 33.0844) -> (-94.9076, 33.0844)
  line L2933 (185.279, 71.1844) -> (185.279, 68.0838)
  line L2934 (238.182, 33.0844) -> (238.182, 38.8844)
  line L2935 (-149.9629, 22.9336) -> (-149.9629, 23.934)
  line L2936 (-95.194, 105.5592) -> (-94.395, 105.5592)
  line L2937 (-163.9637, 23.934) -> (-149.9629, 23.934)
  line L2938 (-94.9076, 38.8844) -> (-94.9076, 33.0844)
  line L2939 (-163.9637, 19.8345) -> (-164.763, 19.8345)
  line L2940 (105.63, 68.0838) -> (104.831, 68.0838)
  line L2941 (-27.72, 108.6602) -> (-27.72, 105.5592)
  line L2942 (16.299, -2.6165) -> (15.473, -2.6165)
  line L2943 (185.279, 80.0836) -> (186.08, 80.0836)
  line L2944 (-94.9076, 42.984) -> (-94.9076, 41.9836)
  line L2945 (-95.708, 29.9838) -> (-95.708, 33.0844)
  line L2946 (-24.269, 105.5592) -> (-23.47, 105.5592)
  line L2947 (111.381, 66.3337) -> (111.381, 67.3134)
  line L2948 (-149.1636, 22.9336) -> (-149.9629, 22.9336)
  line L2949 (-23.47, 108.6602) -> (-23.47, 109.6602)
  line L2950 (186.08, 71.1844) -> (185.279, 71.1844)
  line L2951 (-24.269, 96.6592) -> (-23.47, 96.6592)
  line L2952 (16.299, -2.6165) -> (16.299, 0.1836)
  line L2953 (-95.194, 109.6602) -> (-95.194, 108.6602)
  line L2954 (9.067, 10.9337) -> (9.867, 10.9337)
  line L2955 (238.182, 41.9836) -> (238.182, 42.984)
  line L2956 (-94.501, 120.9832) -> (-95.301, 120.9832)
  line L2957 (243.459, 30.2332) -> (243.459, 31.9583)
  line L2958 (-94.9076, 41.9836) -> (-94.9076, 42.984)
  line L2959 (243.459, 31.9583) -> (243.459, 30.2332)
  line L2960 (185.279, 76.9844) -> (186.08, 76.9844)
  circle A50 centre (-94.901, 117.5832) radius 1.7
  line L2961 (-23.47, 109.6602) -> (-23.47, 108.6602)
  line L2962 (-95.708, 41.9836) -> (-94.9076, 41.9836)
  line L2963 (238.979, 41.9836) -> (238.979, 38.8844)
  line L2964 (-94.395, 108.6602) -> (-95.194, 108.6602)
  line L2965 (-149.9629, 23.934) -> (-163.9637, 23.934)
  line L2966 (-24.269, 108.6602) -> (-23.47, 108.6602)
  line L2967 (185.279, 71.1844) -> (186.08, 71.1844)
  line L2968 (238.979, 29.9838) -> (238.182, 29.9838)
  line L2969 (-90.1451, 105.5592) -> (-90.9441, 105.5592)
  line L2970 (200.082, 80.0836) -> (200.082, 81.084)
  line L2971 (243.459, 35.2589) -> (242.482, 35.2589)
  line L2972 (-149.1636, 22.9336) -> (-149.1636, 19.8345)
  line L2973 (185.279, 80.0836) -> (185.279, 76.9844)
  line L2974 (238.182, 41.9836) -> (238.979, 41.9836)
  line L2975 (-23.47, 96.6592) -> (-23.47, 95.6582)
  line L2976 (-149.9629, 23.934) -> (-149.9629, 22.9336)
  line L2977 (185.279, 76.9844) -> (185.279, 80.0836)
  line L2978 (-99.1575, 29.9838) -> (-99.1575, 33.0844)
  line L2979 (244.232, 38.5083) -> (243.23, 38.5083)
  line L2980 (-99.1575, 29.9838) -> (-99.9579, 29.9838)
  line L2981 (-94.9076, 29.9838) -> (-95.708, 29.9838)
  line L2982 (-90.9441, 108.6602) -> (-90.9441, 105.5592)
  line L2983 (-164.763, 19.8345) -> (-164.763, 22.9336)
  line L2984 (-95.194, 109.6602) -> (-109.1951, 109.6602)
  line L2985 (-23.47, 99.7592) -> (-23.47, 105.5592)
  line L2986 (-90.1451, 108.6602) -> (-90.1451, 109.6602)
  line L2987 (-109.1951, 109.6602) -> (-95.194, 109.6602)
  line L2988 (-99.9579, 29.9838) -> (-99.1575, 29.9838)
  line L2989 (8.724, -8.8866) -> (10.449, -8.8866)
  line L2990 (-163.9637, 22.9336) -> (-163.9637, 23.934)
  arc A51 (-104.601, 120.9832) -> (-106.601, 118.9832) centre (-104.601, 118.9832) ccw
  line L2991 (244.232, 53.3084) -> (244.232, 52.509)
  line L2992 (-99.9579, 33.0844) -> (-99.1575, 33.0844)
  line L2993 (185.279, 68.0838) -> (186.08, 68.0838)
  line L2994 (-42.52, 105.5592) -> (-43.319, 105.5592)
  line L2995 (238.182, 52.1344) -> (238.979, 52.1344)
  line L2996 (-99.1575, 41.9836) -> (-99.9579, 41.9836)
  line L2997 (-109.9941, 108.6602) -> (-109.1951, 108.6602)
  line L2998 (186.08, 81.084) -> (186.08, 80.0836)
  line L2999 (-163.9637, 23.934) -> (-163.9637, 22.9336)
  line L3000 (255.761, 54.0334) -> (252.529, 54.0334)
  line L3001 (-90.1451, 109.6602) -> (-90.1451, 108.6602)
  line L3002 (185.279, 68.0838) -> (185.279, 71.1844)
  line L3003 (13.748, -8.8866) -> (13.748, -9.8664)
  line L3004 (-149.9629, 19.8345) -> (-149.1636, 19.8345)
  line L3005 (186.08, 76.9844) -> (186.08, 71.1844)
  line L3006 (-149.9629, 22.9336) -> (-149.1636, 22.9336)
  line L3007 (10.449, -9.8664) -> (13.748, -9.8664)
  line L3008 (-164.763, 22.9336) -> (-163.9637, 22.9336)
  line L3009 (111.381, 80.5344) -> (111.381, 79.6137)
  line L3010 (247.929, 52.509) -> (247.929, 54.0334)
  line L3011 (10.449, -8.8866) -> (10.449, -9.8664)
  line L3012 (-99.9579, 41.9836) -> (-99.9579, 42.984)
  line L3013 (-164.763, 22.9336) -> (-164.763, 19.8345)
  line L3014 (200.082, 67.0833) -> (200.082, 68.0838)
  line L3015 (8.724, -8.8866) -> (8.724, -4.4162)
  arc A52 (-108.601, 114.1832) -> (-106.601, 116.1832) centre (-108.601, 116.1832) ccw
  line L3016 (104.831, 76.9844) -> (104.831, 76.3836)
  line L3017 (8.724, -4.4162) -> (8.724, -8.8866)
  line L3018 (-95.708, 41.9836) -> (-95.708, 38.8844)
  line L3019 (247.333, 53.3084) -> (244.232, 53.3084)
  line L3020 (-94.395, 105.5592) -> (-94.395, 108.6602)
  line L3021 (243.459, 55.7585) -> (243.459, 54.0334)
  line L3022 (-109.9941, 105.5592) -> (-109.9941, 108.6602)
  line L3023 (-99.1575, 33.0844) -> (-99.1575, 29.9838)
  line L3024 (13.748, -9.8664) -> (13.748, -8.8866)
  line L3025 (-42.52, 108.6602) -> (-42.52, 109.6602)
  line L3026 (-43.319, 105.5592) -> (-43.319, 108.6602)
  line L3027 (10.449, -9.8664) -> (10.449, -8.8866)
  line L3028 (-109.9941, 105.5592) -> (-109.1951, 105.5592)
  line L3029 (-42.52, 52.1344) -> (-43.321, 52.1344)
  line L3030 (186.08, 68.0838) -> (185.279, 68.0838)
  line L3031 (-149.1636, 19.8345) -> (-149.1636, 22.9336)
  line L3032 (113.106, 79.6137) -> (113.106, 76.3836)
  line L3033 (-149.1636, 19.8345) -> (-149.9629, 19.8345)
  line L3034 (18.698, -20.7426) -> (19.498, -20.7426)
  line L3035 (-94.9076, 29.9838) -> (-94.9076, 28.9833)
  line L3036 (252.529, 54.0334) -> (255.761, 54.0334)
  line L3037 (186.08, 80.0836) -> (185.279, 80.0836)
  line L3038 (111.381, 80.5344) -> (108.08, 80.5344)
  line L3039 (-145.2017, 42.984) -> (-159.2012, 42.984)
  line L3040 (186.08, 71.1844) -> (186.08, 76.9844)
  line L3041 (-95.708, 29.9838) -> (-94.9076, 29.9838)
  line L3042 (-94.9076, 33.0844) -> (-94.9076, 38.8844)
  line L3043 (108.08, 80.5344) -> (111.381, 80.5344)
  line L3044 (13.748, -9.8664) -> (10.449, -9.8664)
  line L3045 (108.08, 80.5344) -> (108.08, 79.6137)
  line L3046 (10.449, -8.8866) -> (8.724, -8.8866)
  line L3047 (238.979, 52.1344) -> (238.182, 52.1344)
  line L3048 (-144.4011, 33.0844) -> (-145.2017, 33.0844)
  line L3049 (-43.319, 99.7592) -> (-42.52, 99.7592)
  line L3050 (-144.4011, 29.9838) -> (-145.2017, 29.9838)
  circle A53 centre (19.098, -17.3426) radius 1.7
  line L3051 (-42.52, 99.7592) -> (-43.319, 99.7592)
  line L3052 (-109.1951, 109.6602) -> (-109.1951, 108.6602)
  line L3053 (257.232, 52.509) -> (256.23, 52.509)
  line L3054 (186.08, 67.0833) -> (186.08, 68.0838)
  line L3055 (247.929, 54.0334) -> (243.459, 54.0334)
  line L3056 (200.082, 81.084) -> (200.082, 80.0836)
  line L3057 (-43.319, 99.7592) -> (-43.319, 96.6592)
  line L3058 (-95.708, 38.8844) -> (-94.9076, 38.8844)
  line L3059 (-109.1951, 108.6602) -> (-109.9941, 108.6602)
  circle A54 centre (19.098, -17.3426) radius 1.7
  line L3060 (-95.194, 108.6602) -> (-94.395, 108.6602)
  line L3061 (-159.2012, 28.9833) -> (-145.2017, 28.9833)
  line L3062 (186.08, 80.0836) -> (186.08, 81.084)
  line L3063 (-145.2017, 29.9838) -> (-145.2017, 28.9833)
  line L3064 (-42.52, 95.6582) -> (-42.52, 96.6592)
  line L3065 (186.08, 76.9844) -> (185.279, 76.9844)
  line L3066 (105.63, 76.9844) -> (105.63, 80.0836)
  line L3067 (-94.395, 105.5592) -> (-95.194, 105.5592)
  line L3068 (111.381, 79.6137) -> (113.106, 79.6137)
  line L3069 (-42.52, 61.0336) -> (-43.321, 61.0336)
  line L3070 (-99.9579, 28.9833) -> (-99.9579, 29.9838)
  line L3071 (108.08, 79.6137) -> (108.08, 80.5344)
  line L3072 (242.482, 55.7585) -> (243.459, 55.7585)
  line L3073 (13.748, -8.8866) -> (15.473, -8.8866)
  line L3074 (-145.2017, 28.9833) -> (-145.2017, 29.9838)
  line L3075 (113.93, 73.5836) -> (113.93, 76.3836)
  line L3076 (-106.601, 118.9832) -> (-106.601, 116.1832)
  line L3077 (-145.2017, 33.0844) -> (-145.2017, 38.8844)
  line L3078 (-90.9441, 108.6602) -> (-90.1451, 108.6602)
  line L3079 (-43.319, 96.6592) -> (-43.319, 99.7592)
  line L3080 (256.681, 55.7585) -> (255.761, 55.7585)
  line L3081 (253.129, 53.3084) -> (256.23, 53.3084)
  line L3082 (256.23, 53.3084) -> (256.23, 52.509)
  line L3083 (-43.319, 108.6602) -> (-42.52, 108.6602)
  line L3084 (-99.1575, 41.9836) -> (-99.1575, 38.8844)
  line L3085 (-46.77, 49.0338) -> (-46.77, 52.1344)
  line L3086 (106.355, 76.3836) -> (106.355, 79.6137)
  line L3087 (-42.52, 109.6602) -> (-42.52, 108.6602)
  line L3088 (108.08, 79.6137) -> (106.355, 79.6137)
  line L3089 (253.129, 53.3084) -> (253.129, 52.509)
  line L3090 (-43.321, 61.0336) -> (-42.52, 61.0336)
  line L3091 (-90.9441, 105.5592) -> (-90.1451, 105.5592)
  line L3092 (249.732, 29.4092) -> (252.529, 29.4092)
  line L3093 (-43.321, 52.1344) -> (-42.52, 52.1344)
  line L3094 (15.473, -8.8866) -> (13.748, -8.8866)
  line L3095 (-47.569, 48.0333) -> (-47.569, 49.0338)
  line L3096 (111.381, 79.6137) -> (111.381, 80.5344)
  line L3097 (15.473, -2.6165) -> (15.473, -8.8866)
  line L3098 (-145.2017, 33.0844) -> (-144.4011, 33.0844)
  line L3099 (-109.1951, 105.5592) -> (-109.9941, 105.5592)
  line L3100 (-144.4011, 38.8844) -> (-145.2017, 38.8844)
  line L3101 (-105.233, 19.8345) -> (-105.233, 22.9336)
  line L3102 (-47.569, 61.0336) -> (-47.569, 62.034)
  line L3103 (200.879, 71.1844) -> (200.879, 68.0838)
  line L3104 (-140.1512, -8.1163) -> (-140.9519, -8.1163)
  line L3105 (-28.519, 95.6582) -> (-28.519, 96.6592)
  line L3106 (5.618, 14.0343) -> (4.817, 14.0343)
  line L3107 (-47.569, 52.1344) -> (-46.77, 52.1344)
  line L3108 (-114.244, 109.6602) -> (-114.244, 108.6602)
  line L3109 (-27.72, 99.7592) -> (-28.519, 99.7592)
  line L3110 (252.529, 30.2332) -> (255.761, 30.2332)
  line L3111 (200.879, 71.1844) -> (200.082, 71.1844)
  line L3112 (-28.519, 105.5592) -> (-28.519, 99.7592)
  line L3113 (-90.4329, 23.934) -> (-104.4326, 23.934)
  line L3114 (-113.445, 99.7592) -> (-114.244, 99.7592)
  line L3115 (-140.1512, 3.8837) -> (-140.1512, 4.8841)
  line L3116 (-113.445, 105.5592) -> (-114.244, 105.5592)
  line L3117 (255.761, 36.984) -> (252.529, 36.984)
  line L3118 (255.761, 35.2589) -> (255.761, 36.984)
  line L3119 (204.329, 80.0836) -> (205.13, 80.0836)
  line L3120 (-9.983, 14.0343) -> (-9.983, 10.9337)
  line L3121 (-43.321, 49.0338) -> (-43.321, 52.1344)
  line L3122 (204.329, 71.1844) -> (205.13, 71.1844)
  line L3123 (5.618, 14.0343) -> (5.618, 10.9337)
  line L3124 (-114.244, 108.6602) -> (-113.445, 108.6602)
  line L3125 (-90.4329, 22.9336) -> (-89.6325, 22.9336)
  line L3126 (243.23, 52.509) -> (243.23, 38.5083)
  line L3127 (-14.233, 14.0343) -> (-13.432, 14.0343)
  line L3128 (-140.9519, 3.8837) -> (-140.1512, 3.8837)
  line L3129 (-42.52, 52.1344) -> (-42.52, 57.9344)
  line L3130 (-113.445, 105.5592) -> (-113.445, 108.6602)
  line L3131 (-140.1512, 3.8837) -> (-140.9519, 3.8837)
  line L3132 (5.618, 10.9337) -> (5.618, 14.0343)
  line L3133 (-140.1512, -9.1167) -> (-140.1512, -8.1163)
  line L3134 (4.817, 9.9333) -> (-9.183, 9.9333)
  line L3135 (-14.233, 10.9337) -> (-14.233, 9.9333)
  line L3136 (255.761, 35.2589) -> (256.681, 35.2589)
  line L3137 (-47.569, 62.034) -> (-47.569, 61.0336)
  line L3138 (-28.52, 49.0338) -> (-28.52, 48.0333)
  line L3139 (247.929, 38.5083) -> (247.929, 36.984)
  line L3140 (-114.244, 105.5592) -> (-114.244, 99.7592)
  line L3141 (-13.432, 14.0343) -> (-14.233, 14.0343)
  line L3142 (-28.519, 96.6592) -> (-27.72, 96.6592)
  line L3143 (200.082, 76.9844) -> (200.879, 76.9844)
  line L3144 (-114.244, 96.6592) -> (-113.445, 96.6592)
  line L3145 (-46.77, 61.0336) -> (-46.77, 57.9344)
  line L3146 (-142.5325, 10.9337) -> (-142.5325, 9.9333)
  line L3147 (205.13, 68.0838) -> (205.13, 67.0833)
  line L3148 (247.929, 36.984) -> (247.929, 38.5083)
  line L3149 (252.529, 38.5083) -> (253.129, 38.5083)
  line L3150 (-27.72, 105.5592) -> (-28.519, 105.5592)
  line L3151 (-47.569, 49.0338) -> (-46.77, 49.0338)
  line L3152 (-140.1512, -5.0157) -> (-140.9519, -5.0157)
  line L3153 (-140.1512, -8.1163) -> (-140.1512, -9.1167)
  line L3154 (-43.321, 52.1344) -> (-43.321, 49.0338)
  line L3155 (200.879, 80.0836) -> (200.082, 80.0836)
  line L3156 (-140.1512, 4.8841) -> (-140.1512, 3.8837)
  line L3157 (42.406, 96.6592) -> (43.205, 96.6592)